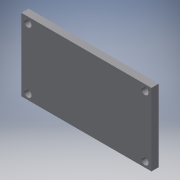
# Autodesk Inventor part: Hoofdplaat onderkant
Saved by Autodesk Inventor 2018.3 (Build 223284000, 284)
## iProperties
Created: 2020-11-23
Part Number: Hoofdplaat onderkant
Material: Generic
Document SubType Name: Modeling
Designer: daanv
Density: 1 g/cm^3
Appearance: Default
Author: daanv
Autodesk Inventor part; units mm, degrees
ref_plane "YZ Plane" through (0, 0, 0) normal (1, 0, 0) x (0, 1, 0)
ref_plane "XZ Plane" through (0, 0, 0) normal (0, 1, 0) x (-1, 0, 0)
ref_plane "XY Plane" through (0, 0, 0) normal (0, 0, 1) x (1, 0, 0)
sketch "Sketch1" plane through (0, 0, 0) normal (0, 0, 1) x (1, 0, 0)
  line L0 (0, 0) -> (90, 0)
  line L1 (90, 0) -> (90, 5)
  line L2 (90, 5) -> (0, 5)
  line L3 (0, 5) -> (0, 0)
  dimension "d0" = 90
  dimension "d1" = 5
  constraints: 8 end point, 2 parallel, 1 horizontal, 1 perpendicular
  measures "d0" distance of L2.end L1.end
  measures "d1" distance of L0.end L1.end
extrude "Extrusion1" add sketch "Sketch1" along normal blind 50
sketch "Sketch2" plane through (0, 5, 0) normal (0, 1, 0) x (1, 0, 0)
  line L0 (90, 0) -> (0, 0) projected
  line L1 (0, 0) -> (0, -50) projected
  line L2 (90, -50) -> (0, -50) projected
  line L3 (90, 0) -> (90, -50) projected
  line L4 (35, -18) -> (55, -18)
  line L5 (55, -18) -> (55, -32)
  line L6 (55, -32) -> (35, -32)
  line L7 (35, -32) -> (35, -18)
  line L8 (53.87, -28.5052) -> (53.2056, -30.55)
  line L9 (53.2056, -30.55) -> (51.0556, -30.55)
  line L10 (51.0556, -30.55) -> (50.3912, -28.5052)
  line L11 (50.3912, -28.5052) -> (52.1306, -27.2415)
  line L12 (52.1306, -27.2415) -> (53.87, -28.5052)
  line L13 (37.8694, -27.2415) -> (39.6088, -28.5052)
  line L14 (39.6088, -28.5052) -> (38.9444, -30.55)
  line L15 (38.9444, -30.55) -> (36.7944, -30.55)
  line L16 (36.7944, -30.55) -> (36.13, -28.5052)
  line L17 (36.13, -28.5052) -> (37.8694, -27.2415)
  line L18 (37.8694, -19.1) -> (39.6088, -20.3637)
  line L19 (39.6088, -20.3637) -> (38.9444, -22.4085)
  line L20 (38.9444, -22.4085) -> (36.7944, -22.4085)
  line L21 (36.7944, -22.4085) -> (36.13, -20.3637)
  line L22 (36.13, -20.3637) -> (37.8694, -19.1)
  line L23 (52.1306, -19.1) -> (53.87, -20.3637)
  line L24 (53.87, -20.3637) -> (53.2056, -22.4085)
  line L25 (53.2056, -22.4085) -> (51.0556, -22.4085)
  line L26 (51.0556, -22.4085) -> (50.3912, -20.3637)
  line L27 (50.3912, -20.3637) -> (52.1306, -19.1)
  point P0 (52.1306, -29.0704)
  point P1 (37.8694, -29.0704)
  point P2 (37.8694, -20.9289)
  point P3 (52.1306, -20.9289)
  point P4 (52.1306, -22.4085)
  dimension "d4" = 20
  dimension "d5" = 14
  dimension "d6" = 18
  dimension "d7" = 18
  dimension "d8" = 35
  dimension "d9" = 35
  dimension "d11" = 1.13
  dimension "d12" = 1.45
  dimension "d13" = 1.45
  dimension "d15" = 1.13
  dimension "d16" = 1.13
  dimension "d17" = 1.1
  dimension "d18" = 1.1
  dimension "d19" = 1.13
  dimension "d28" = 2.15
  dimension "d29" = 2.15
  dimension "d30" = 4.833
  dimension "d31" = 2.15
  dimension "d32" = 2.15
  dimension "d33" = 4.833
  constraints: 48 end point, 4 horizontal, 2 parallel, 1 midpoint, 1 perpendicular, 1 vertical alignment, 44 other
  measures "d4" distance of L5.end L6.end
  measures "d5" distance of L4.end L5.end
  measures "d6" distance between parallel lines of L0 L4
  measures "d7" distance between parallel lines of L2 L6
  measures "d8" distance between parallel lines of L1 L7
  measures "d9" distance between parallel lines of L3 L5
  measures "d11" distance from line of L5 L8.start
  measures "d12" distance between parallel lines of L6 L9
  measures "d13" distance between parallel lines of L6 L15
  measures "d15" distance from line of L7 L16.end
  measures "d16" distance from line of L5 L23.end
  measures "d17" distance from line of L4 L23.start
  measures "d18" distance from line of L4 L18.start
  measures "d19" distance from line of L7 L21.end
  measures "d28" distance of L19.end L20.end
  measures "d29" distance of L14.end L15.end
  measures "d30" distance from line of L13.start L20
  measures "d31" distance of L24.end L25.end
  measures "d32" distance of L8.end L9.end
  measures "d33" distance from line of L11.end L25
extrude "Extrusion2" cut sketch "Sketch2" against normal blind 4.5 contours L8 L9 L10 L11 L12 | L13 L14 L15 L16 L17 | L18 L19 L20 L21 L22 | L23 L24 L25 L26 L27
chamfer "Chamfer1" distance 0.5 angle 45 20 edges at (36.9997, 5, 27.8734) (36.4622, 5, 29.5276) (37.8694, 5, 30.55) (39.2766, 5, 29.5276) (38.7391, 5, 27.8734) (36.9997, 5, 19.7319) (36.4622, 5, 21.3861) (37.8694, 5, 22.4085) (39.2766, 5, 21.3861) (38.7391, 5, 19.7319) (50.7234, 5, 29.5276) (51.2609, 5, 27.8734) (53.0003, 5, 27.8734) (53.5378, 5, 29.5276) (52.1306, 5, 30.55) (52.1306, 5, 22.4085) (50.7234, 5, 21.3861) (51.2609, 5, 19.7319) (53.5378, 5, 21.3861) (53.0003, 5, 19.7319)
sketch "Sketch3" plane through (0, 5, 0) normal (0, 1, 0) x (1, 0, 0)
  line L0 (90, 0) -> (0, 0) projected
  line L1 (90, -50) -> (0, -50) projected
  line L2 (90, 0) -> (90, -50) projected
  line L3 (0, 0) -> (0, -50) projected
  point P0 (4.5, -46)
  point P1 (4.5, -4)
  point P2 (85.5, -46)
  point P3 (85.5, -4)
  dimension "d46" = 4.5
  dimension "d47" = 4.5
  dimension "d48" = 4
  dimension "d49" = 4
  dimension "d57" = 4.5
  dimension "d58" = 4.5
  dimension "d59" = 4
  dimension "d60" = 4
  measures "d46" distance from line of L2 point (85.5, -4)
  measures "d47" distance from line of L2 point (85.5, -46)
  measures "d48" distance from line of L1 point (85.5, -46)
  measures "d49" distance from line of L0 point (85.5, -4)
  measures "d57" distance from line of L3 point (4.5, -46)
  measures "d58" distance from line of L3 point (4.5, -4)
  measures "d59" distance from line of L0 point (4.5, -4)
  measures "d60" distance from line of L1 point (4.5, -46)
hole "Hole2" at (4.5, 5, 46) at (4.5, 5, 4) at (85.5, 5, 4) at (85.5, 5, 46) direction (0, -1, 0) diameter 5 end through all
body "Solid1"
